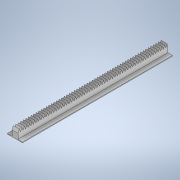
# Autodesk Inventor part: Zahnradbahn_klein
Saved by Autodesk Inventor 2022 (Build 260153000, 153)
## iProperties
Created: 2022-05-05
Part Number: Zahnradbahn_klein
Material: Generisch
Document SubType Name: Modeling
Designer: 123St
Density: 1 g/cm^3
Appearance: Vorgabe
Author: 123St
Autodesk Inventor part; units mm, degrees
ref_plane "YZ Plane" through (0, 0, 0) normal (1, 0, 0) x (0, 1, 0)
ref_plane "XZ Plane" through (0, 0, 0) normal (0, 1, 0) x (-1, 0, 0)
ref_plane "XY Plane" through (0, 0, 0) normal (0, 0, 1) x (1, 0, 0)
sketch "Skizze1" plane through (0, 0, 0) normal (1, 0, 0) x (0, 1, 0)
  line L0 (3.5, 75.65) -> (-3.5, 75.65)
  line L1 (-3.5, 75.65) -> (-3.5, -75.65)
  line L2 (-3.5, -75.65) -> (3.5, -75.65)
  line L3 (3.5, -75.65) -> (3.5, 75.65)
  line L4 (3.5, 75.65) -> (-3.5, -75.65) construction
  line L5 (-3.5, 75.65) -> (3.5, -75.65) construction
  point P0 (0, 0)
  dimension "d0" = 7
  dimension "d1" = 151.3
  constraints: 12 end point, 2 midpoint, 2 parallel, 1 horizontal, 1 perpendicular
  measures "d0" distance of L0.start L0.end
  measures "d1" distance of L2.end L0.start
extrude "Extrusion1" add sketch "Skizze1" along normal blind 4
sketch "Skizze3" plane through (0, -3.5, -75.65) normal (0, -1, 0) x (1, 0, 0)
  line L0 (-3, 151.3) -> (7, 151.3)
  line L1 (7, 151.3) -> (7, 0)
  line L2 (7, 0) -> (-3, 0)
  line L3 (-3, 0) -> (-3, 151.3)
  line L4 (4, 151.3) -> (4, 0) projected
  line L5 (0, 151.3) -> (4, 151.3) projected
  point P0 (0, 75.65)
  dimension "d21" = 151.3
  dimension "d22" = 10
  dimension "d23" = 3
  dimension "d24" = 0
  constraints: 8 end point, 2 parallel, 1 horizontal, 1 perpendicular
  measures "d21" distance of L0.end L1.end
  measures "d22" distance between parallel lines of L3 L1
  measures "d23" distance between parallel lines of L4 L1
  measures "d24" distance between parallel lines of L5 L0
extrude "Extrusion3" add sketch "Skizze3" along normal blind 0.5
sketch "Skizze5" plane through (4, 0, 0) normal (1, 0, 0) x (0, 0, -1)
  line L0 (-75.65, 3.5) -> (-75.65, -3.5) projected
  line L1 (-75.65, 0) -> (-74.8, 2)
  line L2 (-74.8, 2) -> (-73.95, 0)
  line L3 (75.65, 3.5) -> (-75.65, 3.5) projected
  line L4 (-73.1, 2) -> (-72.25, 0)
  line L5 (-73.95, 0) -> (-73.1, 2)
  line L6 (-71.4, 2) -> (-70.55, 0)
  line L7 (-72.25, 0) -> (-71.4, 2)
  line L8 (-69.7, 2) -> (-68.85, 0)
  line L9 (-70.55, 0) -> (-69.7, 2)
  line L10 (-68, 2) -> (-67.15, 0)
  line L11 (-68.85, 0) -> (-68, 2)
  line L12 (-66.3, 2) -> (-65.45, 0)
  line L13 (-67.15, 0) -> (-66.3, 2)
  line L14 (-64.6, 2) -> (-63.75, 0)
  line L15 (-65.45, 0) -> (-64.6, 2)
  line L16 (-62.9, 2) -> (-62.05, 0)
  line L17 (-63.75, 0) -> (-62.9, 2)
  line L18 (-61.2, 2) -> (-60.35, 0)
  line L19 (-62.05, 0) -> (-61.2, 2)
  line L20 (-59.5, 2) -> (-58.65, 0)
  line L21 (-60.35, 0) -> (-59.5, 2)
  line L22 (-57.8, 2) -> (-56.95, 0)
  line L23 (-58.65, 0) -> (-57.8, 2)
  line L24 (-56.1, 2) -> (-55.25, 0)
  line L25 (-56.95, 0) -> (-56.1, 2)
  line L26 (-54.4, 2) -> (-53.55, 0)
  line L27 (-55.25, 0) -> (-54.4, 2)
  line L28 (-52.7, 2) -> (-51.85, 0)
  line L29 (-53.55, 0) -> (-52.7, 2)
  line L30 (-51, 2) -> (-50.15, 0)
  line L31 (-51.85, 0) -> (-51, 2)
  line L32 (-49.3, 2) -> (-48.45, 0)
  line L33 (-50.15, 0) -> (-49.3, 2)
  line L34 (-47.6, 2) -> (-46.75, 0)
  line L35 (-48.45, 0) -> (-47.6, 2)
  line L36 (-45.9, 2) -> (-45.05, 0)
  line L37 (-46.75, 0) -> (-45.9, 2)
  line L38 (-44.2, 2) -> (-43.35, 0)
  line L39 (-45.05, 0) -> (-44.2, 2)
  line L40 (-42.5, 2) -> (-41.65, 0)
  line L41 (-43.35, 0) -> (-42.5, 2)
  line L42 (-40.8, 2) -> (-39.95, 0)
  line L43 (-41.65, 0) -> (-40.8, 2)
  line L44 (-39.1, 2) -> (-38.25, 0)
  line L45 (-39.95, 0) -> (-39.1, 2)
  line L46 (-37.4, 2) -> (-36.55, 0)
  line L47 (-38.25, 0) -> (-37.4, 2)
  line L48 (-35.7, 2) -> (-34.85, 0)
  line L49 (-36.55, 0) -> (-35.7, 2)
  line L50 (-34, 2) -> (-33.15, 0)
  line L51 (-34.85, 0) -> (-34, 2)
  line L52 (-32.3, 2) -> (-31.45, 0)
  line L53 (-33.15, 0) -> (-32.3, 2)
  line L54 (-30.6, 2) -> (-29.75, 0)
  line L55 (-31.45, 0) -> (-30.6, 2)
  line L56 (-28.9, 2) -> (-28.05, 0)
  line L57 (-29.75, 0) -> (-28.9, 2)
  line L58 (-27.2, 2) -> (-26.35, 0)
  line L59 (-28.05, 0) -> (-27.2, 2)
  line L60 (-25.5, 2) -> (-24.65, 0)
  line L61 (-26.35, 0) -> (-25.5, 2)
  line L62 (-23.8, 2) -> (-22.95, 0)
  line L63 (-24.65, 0) -> (-23.8, 2)
  line L64 (-22.1, 2) -> (-21.25, 0)
  line L65 (-22.95, 0) -> (-22.1, 2)
  line L66 (-20.4, 2) -> (-19.55, 0)
  line L67 (-21.25, 0) -> (-20.4, 2)
  line L68 (-18.7, 2) -> (-17.85, 0)
  line L69 (-19.55, 0) -> (-18.7, 2)
  line L70 (-17, 2) -> (-16.15, 0)
  line L71 (-17.85, 0) -> (-17, 2)
  line L72 (-15.3, 2) -> (-14.45, 0)
  line L73 (-16.15, 0) -> (-15.3, 2)
  line L74 (-13.6, 2) -> (-12.75, 0)
  line L75 (-14.45, 0) -> (-13.6, 2)
  line L76 (-11.9, 2) -> (-11.05, 0)
  line L77 (-12.75, 0) -> (-11.9, 2)
  line L78 (-10.2, 2) -> (-9.35, 0)
  line L79 (-11.05, 0) -> (-10.2, 2)
  line L80 (-8.5, 2) -> (-7.65, 0)
  line L81 (-9.35, 0) -> (-8.5, 2)
  line L82 (-6.8, 2) -> (-5.95, 0)
  line L83 (-7.65, 0) -> (-6.8, 2)
  line L84 (-5.1, 2) -> (-4.25, 0)
  line L85 (-5.95, 0) -> (-5.1, 2)
  line L86 (-3.4, 2) -> (-2.55, 0)
  line L87 (-4.25, 0) -> (-3.4, 2)
  line L88 (-1.7, 2) -> (-0.85, 0)
  line L89 (-2.55, 0) -> (-1.7, 2)
  line L90 (0, 2) -> (0.85, 0)
  line L91 (-0.85, 0) -> (0, 2)
  line L92 (1.7, 2) -> (2.55, 0)
  line L93 (0.85, 0) -> (1.7, 2)
  line L94 (3.4, 2) -> (4.25, 0)
  line L95 (2.55, 0) -> (3.4, 2)
  line L96 (5.1, 2) -> (5.95, 0)
  line L97 (4.25, 0) -> (5.1, 2)
  line L98 (6.8, 2) -> (7.65, 0)
  line L99 (5.95, 0) -> (6.8, 2)
  line L100 (8.5, 2) -> (9.35, 0)
  line L101 (7.65, 0) -> (8.5, 2)
  line L102 (10.2, 2) -> (11.05, 0)
  line L103 (9.35, 0) -> (10.2, 2)
  line L104 (11.9, 2) -> (12.75, 0)
  line L105 (11.05, 0) -> (11.9, 2)
  line L106 (13.6, 2) -> (14.45, 0)
  line L107 (12.75, 0) -> (13.6, 2)
  line L108 (15.3, 2) -> (16.15, 0)
  line L109 (14.45, 0) -> (15.3, 2)
  line L110 (17, 2) -> (17.85, 0)
  line L111 (16.15, 0) -> (17, 2)
  line L112 (18.7, 2) -> (19.55, 0)
  line L113 (17.85, 0) -> (18.7, 2)
  line L114 (20.4, 2) -> (21.25, 0)
  line L115 (19.55, 0) -> (20.4, 2)
  line L116 (22.1, 2) -> (22.95, 0)
  line L117 (21.25, 0) -> (22.1, 2)
  line L118 (23.8, 2) -> (24.65, 0)
  line L119 (22.95, 0) -> (23.8, 2)
  line L120 (25.5, 2) -> (26.35, 0)
  line L121 (24.65, 0) -> (25.5, 2)
  line L122 (27.2, 2) -> (28.05, 0)
  line L123 (26.35, 0) -> (27.2, 2)
  line L124 (28.9, 2) -> (29.75, 0)
  line L125 (28.05, 0) -> (28.9, 2)
  line L126 (30.6, 2) -> (31.45, 0)
  line L127 (29.75, 0) -> (30.6, 2)
  line L128 (32.3, 2) -> (33.15, 0)
  line L129 (31.45, 0) -> (32.3, 2)
  line L130 (34, 2) -> (34.85, 0)
  line L131 (33.15, 0) -> (34, 2)
  line L132 (35.7, 2) -> (36.55, 0)
  line L133 (34.85, 0) -> (35.7, 2)
  line L134 (37.4, 2) -> (38.25, 0)
  line L135 (36.55, 0) -> (37.4, 2)
  line L136 (39.1, 2) -> (39.95, 0)
  line L137 (38.25, 0) -> (39.1, 2)
  line L138 (40.8, 2) -> (41.65, 0)
  line L139 (39.95, 0) -> (40.8, 2)
  line L140 (42.5, 2) -> (43.35, 0)
  line L141 (41.65, 0) -> (42.5, 2)
  line L142 (44.2, 2) -> (45.05, 0)
  line L143 (43.35, 0) -> (44.2, 2)
  line L144 (45.9, 2) -> (46.75, 0)
  line L145 (45.05, 0) -> (45.9, 2)
  line L146 (47.6, 2) -> (48.45, 0)
  line L147 (46.75, 0) -> (47.6, 2)
  line L148 (49.3, 2) -> (50.15, 0)
  line L149 (48.45, 0) -> (49.3, 2)
  line L150 (51, 2) -> (51.85, 0)
  line L151 (50.15, 0) -> (51, 2)
  line L152 (52.7, 2) -> (53.55, 0)
  line L153 (51.85, 0) -> (52.7, 2)
  line L154 (54.4, 2) -> (55.25, 0)
  line L155 (53.55, 0) -> (54.4, 2)
  line L156 (56.1, 2) -> (56.95, 0)
  line L157 (55.25, 0) -> (56.1, 2)
  line L158 (57.8, 2) -> (58.65, 0)
  line L159 (56.95, 0) -> (57.8, 2)
  line L160 (59.5, 2) -> (60.35, 0)
  line L161 (58.65, 0) -> (59.5, 2)
  line L162 (61.2, 2) -> (62.05, 0)
  line L163 (60.35, 0) -> (61.2, 2)
  line L164 (62.9, 2) -> (63.75, 0)
  line L165 (62.05, 0) -> (62.9, 2)
  line L166 (64.6, 2) -> (65.45, 0)
  line L167 (63.75, 0) -> (64.6, 2)
  line L168 (66.3, 2) -> (67.15, 0)
  line L169 (65.45, 0) -> (66.3, 2)
  line L170 (68, 2) -> (68.85, 0)
  line L171 (67.15, 0) -> (68, 2)
  line L172 (69.7, 2) -> (70.55, 0)
  line L173 (68.85, 0) -> (69.7, 2)
  line L174 (71.4, 2) -> (72.25, 0)
  line L175 (70.55, 0) -> (71.4, 2)
  line L176 (73.1, 2) -> (73.95, 0)
  line L177 (72.25, 0) -> (73.1, 2)
  line L178 (74.8, 2) -> (75.65, 0)
  line L179 (73.95, 0) -> (74.8, 2)
  line L180 (76.5, 2) -> (77.35, 0)
  line L181 (75.65, 0) -> (76.5, 2)
  line L182 (78.2, 2) -> (79.05, 0)
  line L183 (77.35, 0) -> (78.2, 2)
  line L184 (79.9, 2) -> (80.75, 0)
  line L185 (79.05, 0) -> (79.9, 2)
  line L186 (81.6, 2) -> (82.45, 0)
  line L187 (80.75, 0) -> (81.6, 2)
  line L188 (83.3, 2) -> (84.15, 0)
  line L189 (82.45, 0) -> (83.3, 2)
  line L190 (85, 2) -> (85.85, 0)
  line L191 (84.15, 0) -> (85, 2)
  line L192 (86.7, 2) -> (87.55, 0)
  line L193 (85.85, 0) -> (86.7, 2)
  line L194 (88.4, 2) -> (89.25, 0)
  line L195 (87.55, 0) -> (88.4, 2)
  line L196 (90.1, 2) -> (90.95, 0)
  line L197 (89.25, 0) -> (90.1, 2)
  line L198 (91.8, 2) -> (92.65, 0)
  line L199 (90.95, 0) -> (91.8, 2)
  line L200 (93.5, 2) -> (94.35, 0)
  line L201 (92.65, 0) -> (93.5, 2)
  line L202 (95.2, 2) -> (96.05, 0)
  line L203 (94.35, 0) -> (95.2, 2)
  line L204 (96.9, 2) -> (97.75, 0)
  line L205 (96.05, 0) -> (96.9, 2)
  line L206 (98.6, 2) -> (99.45, 0)
  line L207 (97.75, 0) -> (98.6, 2)
  line L208 (100.3, 2) -> (101.15, 0)
  line L209 (99.45, 0) -> (100.3, 2)
  line L210 (102, 2) -> (102.85, 0)
  line L211 (101.15, 0) -> (102, 2)
  line L212 (103.7, 2) -> (104.55, 0)
  line L213 (102.85, 0) -> (103.7, 2)
  line L214 (105.4, 2) -> (106.25, 0)
  line L215 (104.55, 0) -> (105.4, 2)
  line L216 (107.1, 2) -> (107.95, 0)
  line L217 (106.25, 0) -> (107.1, 2)
  line L218 (108.8, 2) -> (109.65, 0)
  line L219 (107.95, 0) -> (108.8, 2)
  line L220 (110.5, 2) -> (111.35, 0)
  line L221 (109.65, 0) -> (110.5, 2)
  line L222 (112.2, 2) -> (113.05, 0)
  line L223 (111.35, 0) -> (112.2, 2)
  line L224 (113.9, 2) -> (114.75, 0)
  line L225 (113.05, 0) -> (113.9, 2)
  line L226 (115.6, 2) -> (116.45, 0)
  line L227 (114.75, 0) -> (115.6, 2)
  line L228 (117.3, 2) -> (118.15, 0)
  line L229 (116.45, 0) -> (117.3, 2)
  line L230 (119, 2) -> (119.85, 0)
  line L231 (118.15, 0) -> (119, 2)
  line L232 (120.7, 2) -> (121.55, 0)
  line L233 (119.85, 0) -> (120.7, 2)
  line L234 (122.4, 2) -> (123.25, 0)
  line L235 (121.55, 0) -> (122.4, 2)
  line L236 (124.1, 2) -> (124.95, 0)
  line L237 (123.25, 0) -> (124.1, 2)
  line L238 (125.8, 2) -> (126.65, 0)
  line L239 (124.95, 0) -> (125.8, 2)
  line L240 (127.5, 2) -> (128.35, 0)
  line L241 (126.65, 0) -> (127.5, 2)
  line L242 (129.2, 2) -> (130.05, 0)
  line L243 (128.35, 0) -> (129.2, 2)
  line L244 (130.9, 2) -> (131.75, 0)
  line L245 (130.05, 0) -> (130.9, 2)
  line L246 (132.6, 2) -> (133.45, 0)
  line L247 (131.75, 0) -> (132.6, 2)
  line L248 (134.3, 2) -> (135.15, 0)
  line L249 (133.45, 0) -> (134.3, 2)
  line L250 (136, 2) -> (136.85, 0)
  line L251 (135.15, 0) -> (136, 2)
  line L252 (-75.65, 3.5) -> (-75.65, -3.5) projected
  line L253 (-75.65, 0) -> (-75.65, 3.5)
  line L254 (-75.65, 3.5) -> (75.65, 3.5)
  line L255 (75.65, -3.5) -> (75.65, 3.5) projected
  line L256 (121.55, 0) -> (75.65, 3.5)
  point P0 (0, 0)
  point P1 (119.85, 0)
  point P2 (-73.95, 0)
  point P3 (-72.25, 0)
  point P4 (-70.55, 0)
  point P5 (-68.85, 0)
  point P6 (-67.15, 0)
  point P7 (-65.45, 0)
  point P8 (-63.75, 0)
  point P9 (-62.05, 0)
  point P10 (-60.35, 0)
  point P11 (-58.65, 0)
  point P12 (-56.95, 0)
  point P13 (-55.25, 0)
  point P14 (-53.55, 0)
  point P15 (-51.85, 0)
  point P16 (-50.15, 0)
  point P17 (-48.45, 0)
  point P18 (-46.75, 0)
  point P19 (-45.05, 0)
  point P20 (-43.35, 0)
  point P21 (-41.65, 0)
  point P22 (-39.95, 0)
  point P23 (-38.25, 0)
  point P24 (-36.55, 0)
  point P25 (-34.85, 0)
  point P26 (-33.15, 0)
  point P27 (-31.45, 0)
  point P28 (-29.75, 0)
  point P29 (-28.05, 0)
  point P30 (-26.35, 0)
  point P31 (-24.65, 0)
  point P32 (-22.95, 0)
  point P33 (-21.25, 0)
  point P34 (-19.55, 0)
  point P35 (-17.85, 0)
  point P36 (-16.15, 0)
  point P37 (-14.45, 0)
  point P38 (-12.75, 0)
  point P39 (-11.05, 0)
  point P40 (-9.35, 0)
  point P41 (-7.65, 0)
  point P42 (-5.95, 0)
  point P43 (-4.25, 0)
  point P44 (-2.55, 0)
  point P45 (-0.85, 0)
  point P46 (0.85, 0)
  point P47 (2.55, 0)
  point P48 (4.25, 0)
  point P49 (5.95, 0)
  point P50 (7.65, 0)
  point P51 (9.35, 0)
  point P52 (11.05, 0)
  point P53 (12.75, 0)
  point P54 (14.45, 0)
  point P55 (16.15, 0)
  point P56 (17.85, 0)
  point P57 (19.55, 0)
  point P58 (21.25, 0)
  point P59 (22.95, 0)
  point P60 (24.65, 0)
  point P61 (26.35, 0)
  point P62 (28.05, 0)
  point P63 (29.75, 0)
  point P64 (31.45, 0)
  point P65 (33.15, 0)
  point P66 (34.85, 0)
  point P67 (36.55, 0)
  point P68 (38.25, 0)
  point P69 (39.95, 0)
  point P70 (41.65, 0)
  point P71 (43.35, 0)
  point P72 (45.05, 0)
  point P73 (46.75, 0)
  point P74 (48.45, 0)
  point P75 (50.15, 0)
  point P76 (51.85, 0)
  point P77 (53.55, 0)
  point P78 (55.25, 0)
  point P79 (56.95, 0)
  point P80 (58.65, 0)
  point P81 (60.35, 0)
  point P82 (62.05, 0)
  point P83 (63.75, 0)
  point P84 (65.45, 0)
  point P85 (67.15, 0)
  point P86 (68.85, 0)
  point P87 (70.55, 0)
  point P88 (72.25, 0)
  point P89 (73.95, 0)
  point P90 (75.65, 0)
  point P91 (77.35, 0)
  point P92 (79.05, 0)
  point P93 (80.75, 0)
  point P94 (82.45, 0)
  point P95 (84.15, 0)
  point P96 (85.85, 0)
  point P97 (87.55, 0)
  point P98 (89.25, 0)
  point P99 (90.95, 0)
  point P100 (92.65, 0)
  point P101 (94.35, 0)
  point P102 (96.05, 0)
  point P103 (97.75, 0)
  point P104 (99.45, 0)
  point P105 (101.15, 0)
  point P106 (102.85, 0)
  point P107 (104.55, 0)
  point P108 (106.25, 0)
  point P109 (107.95, 0)
  point P110 (109.65, 0)
  point P111 (111.35, 0)
  point P112 (113.05, 0)
  point P113 (114.75, 0)
  point P114 (116.45, 0)
  point P115 (118.15, 0)
  point P116 (75.65, 0)
  point P117 (83.5152, 3.0934)
  point P118 (121.55, 0)
  point P119 (119.9034, 0.1256)
  point P120 (119.7931, 0.134)
  point P121 (118.2567, 0.2511)
  point P122 (118.0361, 0.2679)
  point P123 (116.6101, 0.3767)
  point P124 (116.2792, 0.4019)
  point P125 (114.9635, 0.5022)
  point P126 (114.5222, 0.5359)
  point P127 (113.3168, 0.6278)
  point P128 (112.7653, 0.6699)
  point P129 (111.6702, 0.7534)
  point P130 (111.0084, 0.8038)
  point P131 (110.0235, 0.8789)
  point P132 (109.2514, 0.9378)
  point P133 (108.3769, 1.0045)
  point P134 (107.4945, 1.0718)
  point P135 (106.7303, 1.13)
  point P136 (105.7376, 1.2057)
  point P137 (105.0836, 1.2556)
  point P138 (103.9806, 1.3397)
  point P139 (103.437, 1.3812)
  point P140 (102.2237, 1.4737)
  point P141 (101.7904, 1.5067)
  point P142 (100.4667, 1.6077)
  point P143 (100.1437, 1.6323)
  point P144 (98.7098, 1.7416)
  point P145 (98.4971, 1.7578)
  point P146 (96.9529, 1.8756)
  point P147 (96.8504, 1.8834)
  point P148 (95.3517, 1.9961)
  point P149 (95.3484, 1.9963)
  point P150 (93.8315, 2.3083)
  point P151 (93.6729, 2.3186)
  point P152 (92.0834, 2.4213)
  point P153 (92.0184, 2.4255)
  point P154 (90.4829, 2.6873)
  point P155 (90.2231, 2.7013)
  point P156 (88.743, 2.7811)
  point P157 (88.5611, 2.7909)
  point P158 (87.0032, 2.8748)
  point P159 (86.8992, 2.8804)
  point P160 (85.2634, 2.9686)
  point P161 (85.2372, 2.97)
  point P162 (83.5863, 3.0899)
  point P163 (75.65, 0)
  dimension "d34" = 1.7
  dimension "d35" = 0.85
  dimension "d38" = 1.7
  dimension "d46" = 2
  dimension "d47" = 3.5
  dimension "d48" = 0
  constraints: 504 end point, 1 horizontal, 1 midpoint, 1 perpendicular, 1 vertical, 624 other
  measures "d34" distance of L1.start L2.end
  measures "d35" horizontal distance of L2.end L1.end
  measures "d38" distance of L1.end L4.start
  measures "d46" vertical distance of L1.start L1.end
  measures "d47" distance from line of L3 L1.start
  measures "d48" vertical distance of L1.start L2.end
extrude "Extrusion5" cut sketch "Skizze5" against normal blind 10 contours L3 L255 L178 L179 L176 L177 L174 L175 L172 L173 L170 L171 L168 L169 L166 L167 L164 L165 L162 L163 L160 L161 L158 L159 L156 L157 L154 L155 L152 L153 L150 L151 L148 L149 L146 L147 L144 L145 L142 L143 L140 L141 L138 L139 L136 L137 L134 L135 L132 L133 L130 L131 L128 L129 L126 L127 L124 L125 L122 L123 L120 L121 L118 L119 L116 L117 L114 L115 L112 L113 L110 L111 L108 L109 L106 L107 L104 L105 L102 L103 L100 L101 L98 L99 L96 L97 L94 L95 L92 L93 L90 L91 L88 L89 L86 L87 L84 L85 L82 L83 L80 L81 L78 L79 L76 L77 L74 L75 L72 L73 L70 L71 L68 L69 L66 L67 L64 L65 L62 L63 L60 L61 L58 L59 L56 L57 L54 L55 L52 L53 L50 L51 L48 L49 L46 L47 L44 L45 L42 L43 L40 L41 L38 L39 L36 L37 L34 L35 L32 L33 L30 L31 L28 L29 L26 L27 L24 L25 L22 L23 L20 L21 L18 L19 L16 L17 L14 L15 L12 L13 L10 L11 L8 L9 L6 L7 L4 L5 L2 L1 L0 | L256 L233 L230 | L256 L231 L228 | L256 L229 L226 | L256 L227 L224 | L256 L225 L222 | L256 L223 L220 | L256 L221 L218 | L256 L219 L216 | L256 L217 L214 | L256 L215 L212 | L256 L213 L210 | L256 L211 L208 | L256 L209 L206 | L256 L207 L204
sketch "Skizze4" plane through (7, -3.5, 75.65) normal (1, 0, 0) x (0, 0, -1)
  line L0 (159.798, 12.6836) -> (48.4645, 12.6836)
  line L1 (48.4645, 12.6836) -> (48.4645, -7.7347)
  line L2 (48.4645, -7.7347) -> (159.798, -7.7347)
  line L3 (159.798, -7.7347) -> (159.798, 12.6836)
  point P0 (75.65, 3.5)
  constraints: 8 end point, 2 parallel, 1 horizontal, 1 perpendicular
extrude "Extrusion4" [suppressed]
sketch "Skizze6" plane through (7, -3.5, 75.65) normal (1, 0, 0) x (0, 0, -1)
  line L0 (156.3463, 21.6609) -> (100, 21.6609)
  line L1 (100, 21.6609) -> (100, -20.81)
  line L2 (100, -20.81) -> (156.3463, -20.81)
  line L3 (156.3463, -20.81) -> (156.3463, 21.6609)
  line L4 (0, 3.5) -> (0, 0) projected
  point P0 (75.65, 3.5)
  dimension "d49" = 100
  constraints: 8 end point, 2 parallel, 1 horizontal, 1 perpendicular
  measures "d49" distance between parallel lines of L4 L1
extrude "Extrusion6" cut sketch "Skizze6" against normal blind 10
